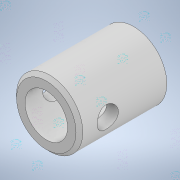
# Autodesk Inventor part: Ch7(5) Part 5 Sleeve
Saved by Autodesk Inventor 2020 (Build 240168000, 168)
## iProperties
Created: 2021-03-04
Part Number: Ch7(5) Part 5 Sleeve
Material: Generic
Document SubType Name: Modeling
Designer: adriggs
Density: 1 g/cm^3
Appearance: Default
Author: adriggs
Autodesk Inventor part; units mm, degrees
ref_plane "YZ Plane" through (0, 0, 0) normal (1, 0, 0) x (0, 1, 0)
ref_plane "XZ Plane" through (0, 0, 0) normal (0, 1, 0) x (-1, 0, 0)
ref_plane "XY Plane" through (0, 0, 0) normal (0, 0, 1) x (1, 0, 0)
sketch "Sketch1" plane through (0, 0, 0) normal (0, 0, 1) x (1, 0, 0)
  line L0 (-20.7493, 0) -> (20.7493, 0) projected
  line L1 (0, -20.7493) -> (0, 20.7493) projected
  circle A0 centre (0, 0) radius 14.8209
  circle A1 centre (0, 0) radius 9.525
  dimension "d2" = 29.6418
  dimension "d3" = 19.05
  constraints: 2 centre point, 2 coincident
  measures "d2" diameter of A0
  measures "d3" diameter of A1
extrude "Extrusion1" add sketch "Sketch1" against normal blind 39.116 contours A1 L1 A0 L0 | L0 A0 L1 A1 | A1 L0 A0 L1 | L1 A0 L0 A1
chamfer "Chamfer1" distance 1.524 angle 45 1 edges at (-14.8209, 0, 0) measured on face at (14.7728, -1.1926, -26.0773)
sketch "Sketch2" plane through (0, 0, 0) normal (1, 0, 0) x (0, 1, 0)
  line L0 (-14.8209, -39.116) -> (14.8209, -39.116) projected
  line L1 (14.8209, -1.524) -> (14.8209, -39.116) projected
  circle A0 centre (0, -12.7) radius 4.7625
  point P0 (0, 0)
  dimension "d9" = 26.416
  dimension "d10" = 9.525
  constraints: 1 centre point, 1 coincident, 1 vertical alignment
  measures "d9" vertical distance of L0.end point (0, -12.7)
  measures "d10" diameter of A0
extrude "Extrusion2" cut sketch "Sketch2" along normal through all both and the other way through all
body "Solid1"
